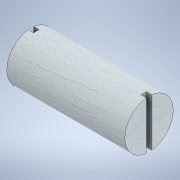
# Autodesk Inventor part: Conveyor Belt Shaft
Saved by Autodesk Inventor 2022.2 (Build 262287000, 287)
## iProperties
Created: 2022-02-21
Part Number: Conveyor Belt Shaft
Material: Stainless Steel AISI 440C, Welded
Document SubType Name: Modeling
Designer: PRASHANTH
Density: 7.8 g/cm^3
Appearance: Wood - Painted White
Author: PRASHANTH
Autodesk Inventor part; units mm, degrees
ref_plane "YZ Plane" through (0, 0, 0) normal (1, 0, 0) x (0, 1, 0)
ref_plane "XZ Plane" through (0, 0, 0) normal (0, 1, 0) x (-1, 0, 0)
ref_plane "XY Plane" through (0, 0, 0) normal (0, 0, 1) x (1, 0, 0)
sketch "Sketch1" plane through (0, 0, 0) normal (1, 0, 0) x (0, 1, 0)
  circle A0 centre (0, 0) radius 22.5
  dimension "d0" = 45
  constraints: 1 centre point, 1 coincident
  measures "d0" diameter of A0
extrude "Extrusion1" add sketch "Sketch1" along normal blind 110
sketch "Sketch2" plane through (110, 0, 0) normal (1, 0, 0) x (0, 0, -1)
  line L0 (2.5, 26.6733) -> (-2.5, 26.6733)
  line L1 (-2.5, 26.6733) -> (-2.5, -26.6733)
  line L2 (-2.5, -26.6733) -> (2.5, -26.6733)
  line L3 (2.5, -26.6733) -> (2.5, 26.6733)
  line L4 (2.5, 26.6733) -> (-2.5, -26.6733) construction
  line L5 (-2.5, 26.6733) -> (2.5, -26.6733) construction
  circle A0 centre (0, 0) radius 2.5
  dimension "d3" = 5
  dimension "d12" = 5
  constraints: 12 end point, 2 midpoint, 2 parallel, 1 centre point, 1 coincident, 1 horizontal, 1 perpendicular
  measures "d3" distance of L0.start L0.end
  measures "d12" diameter of A0
extrude "Extrusion2" cut sketch "Sketch2" against normal blind 5
sketch "Sketch4" plane through (0, 0, 0) normal (-1, 0, 0) x (0, 0, 1)
  line L0 (-2.5, -27.3209) -> (2.5, -27.3209)
  line L1 (2.5, -27.3209) -> (2.5, 27.3209)
  line L2 (2.5, 27.3209) -> (-2.5, 27.3209)
  line L3 (-2.5, 27.3209) -> (-2.5, -27.3209)
  line L4 (-2.5, -27.3209) -> (2.5, 27.3209) construction
  line L5 (2.5, -27.3209) -> (-2.5, 27.3209) construction
  point P0 (0, 0)
  dimension "d9" = 5
  constraints: 12 end point, 2 midpoint, 2 parallel, 1 horizontal, 1 perpendicular
  measures "d9" distance of L2.end L1.end
extrude "Extrusion4" cut sketch "Sketch4" against normal blind 5
sketch "Sketch5" plane through (105, 0, 0) normal (1, 0, 0) x (0, 0, -1)
  circle A0 centre (0, 0) radius 2.5
  dimension "d13" = 5
  constraints: 1 centre point, 1 coincident
  measures "d13" diameter of A0
extrude "Extrusion5" cut sketch "Sketch5" against normal blind 90
body "Solid1"
